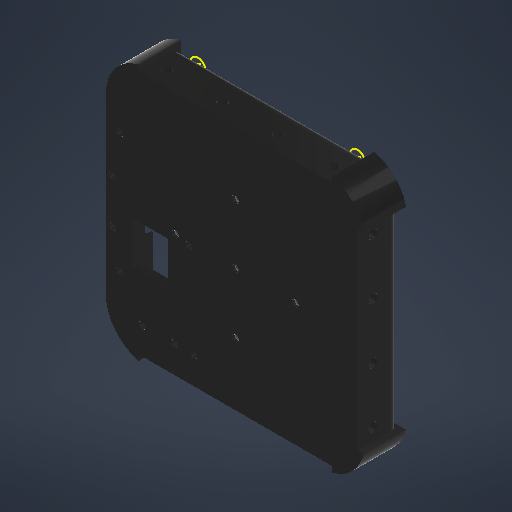
# Autodesk Inventor part: battery_spacer
Saved by Autodesk Inventor 2026.1 (Build 301233000, 233)
## iProperties
Created: 2026-05-19
Part Number: battery_spacer
Material: ABS Plastic
Document SubType Name: Modeling
Designer: aaron
Density: 1.06 g/cm^3
Appearance: Smooth - White
Author: aaron
Autodesk Inventor part; units mm, degrees
ref_plane "YZ Plane" through (0, 0, 0) normal (1, 0, 0) x (0, 1, 0)
ref_plane "XZ Plane" through (0, 0, 0) normal (0, 1, 0) x (-1, 0, 0)
ref_plane "XY Plane" through (0, 0, 0) normal (0, 0, 1) x (1, 0, 0)
sketch "Sketch1" plane through (0, 0, 0) normal (0, 0, 1) x (1, 0, 0)
  circle A0 centre (-25.1008, -25.8499) radius 6
  circle A1 centre (30.8992, 30.1501) radius 6
  circle A2 centre (56.8992, 30.1501) radius 2.15
  circle A3 centre (-51.1008, -25.8499) radius 2.15
  circle A4 centre (-51.1008, 30.1501) radius 2.15
  circle A5 centre (56.8992, -25.8499) radius 2.15
  circle A6 centre (30.8992, 56.1501) radius 2.15
  circle A7 centre (-25.1008, -51.8499) radius 2.15
  circle A8 centre (-25.1008, 56.1501) radius 2.15
  circle A9 centre (30.8992, -51.8499) radius 2.15
  line L0 (48.0316, -57.806) -> (48.0316, -55.1499)
  arc A10 (48.0316, -57.806) -> (62.8553, -42.9824) centre (43.3992, -38.3499) ccw
  line L1 (60.1992, -42.9824) -> (62.8553, -42.9824)
  line L2 (60.1992, -42.9824) -> (60.1992, 47.2825)
  line L3 (62.8553, 47.2825) -> (60.1992, 47.2825)
  arc A11 (62.8553, 47.2825) -> (48.0316, 62.1062) centre (43.3992, 42.6501) ccw
  line L4 (48.0316, 59.4501) -> (48.0316, 62.1062)
  line L5 (48.0316, 59.4501) -> (-42.2333, 59.4501)
  line L6 (-42.2333, 62.1062) -> (-42.2333, 59.4501)
  arc A12 (-42.2333, 62.1062) -> (-57.6008, 42.6501) centre (-37.6008, 42.6501) ccw
  line L7 (-57.6008, -38.3499) -> (-57.6008, 42.6501)
  arc A13 (-57.6008, -38.3499) -> (-42.2333, -57.806) centre (-37.6008, -38.3499) ccw
  line L8 (-42.2333, -55.1499) -> (-42.2333, -57.806)
  line L9 (-42.2333, -55.1499) -> (48.0316, -55.1499)
  circle A14 centre (-25.1008, 2.1501) radius 2.15
  circle A15 centre (2.8992, 30.1501) radius 2.15
  circle A16 centre (30.8992, 2.1501) radius 2.15
  circle A17 centre (2.8992, -25.8499) radius 2.15
  circle A18 centre (2.8992, 2.1501) radius 2.15
  circle A19 centre (-39.1008, -39.8499) radius 13.125
  circle A20 centre (-11.1008, -39.8499) radius 13.125
  circle A21 centre (-11.1008, 16.1501) radius 13.125
  circle A22 centre (44.8992, 16.1501) radius 13.125
  circle A23 centre (44.8992, -11.8499) radius 13.125
  circle A24 centre (44.8992, -39.8499) radius 13.125
  circle A25 centre (16.8992, 44.1501) radius 13.125
  circle A26 centre (16.8992, 16.1501) radius 13.125
  circle A27 centre (16.8992, -11.8499) radius 13.125
  circle A28 centre (16.8992, -39.8499) radius 13.125
  circle A29 centre (-11.1008, 44.1501) radius 13.125
  circle A30 centre (-11.1008, -11.8499) radius 13.125
  circle A31 centre (-39.1008, 44.1501) radius 13.125
  circle A32 centre (-39.1008, -11.8499) radius 13.125
  circle A33 centre (44.8992, 44.1501) radius 13.125
  circle A34 centre (30.8992, -25.8499) radius 6
  circle A35 centre (-25.1008, 30.1501) radius 6
  point P0 (0, 0)
  point P1 (54.9491, 53.8254)
  constraints: 36 centre point, 20 end point, 8 point on circle
extrude "Extrusion1" add sketch "Sketch1" along normal blind 19.82 contours A0 | A1 | A2 | A3 | A4 | A5 | A6 | A7 | A8 | A9 | L0 L9 L8 A13 L7 A12 L6 L5 L4 A11 L3 L2 L1 A10 | A14 | A15 | A16 | A17 | A18 | A19 | A20 | A21 | A22 | A23 | A24 | A25 | A26 | A27 | A28 | A29 | A30 | A31 | A32 | A33 | A34 | A35
fillet "Fillet1" radius 5 3 edges at (2.8992, 59.4501, 0) (2.8992, -55.1499, 0) (60.1992, 2.1501, 0)
sketch "Sketch2" plane through (-42.2333, 59.4501, 19.82) normal (0, 1, 0) x (1, 0, 0)
  circle A0 centre (6.1325, 7) radius 1.65 projected
  circle A1 centre (32.1325, 7) radius 1.65 projected
  circle A2 centre (58.1325, 7) radius 1.65 projected
  circle A3 centre (84.1325, 7) radius 1.65 projected
  circle A4 centre (6.1325, 7) radius 2.15
  circle A5 centre (32.1325, 7) radius 2.15
  circle A6 centre (58.1325, 7) radius 2.15
  circle A7 centre (84.1325, 7) radius 2.15
  point P0 (42.2333, 19.82)
  dimension "d3" = 4.3
  dimension "d4" = 4.3
  dimension "d5" = 4.3
  dimension "d6" = 4.3
  constraints: 4 centre point, 4 coincident
  measures "d3" diameter of A4
  measures "d4" diameter of A5
  measures "d5" diameter of A6
  measures "d6" diameter of A7
sketch "Sketch3" plane through (60.1992, -42.9824, 19.82) normal (1, 0, 0) x (0, 0, -1)
  circle A0 centre (7, 84.1125) radius 1.65 projected
  circle A1 centre (7, 58.1125) radius 1.65 projected
  circle A2 centre (7, 32.1125) radius 1.65 projected
  circle A3 centre (7, 6.1125) radius 1.65 projected
  circle A4 centre (7, 6.1125) radius 2.15
  circle A5 centre (7, 32.1125) radius 2.15
  circle A6 centre (7, 58.1125) radius 2.15
  circle A7 centre (7, 84.1125) radius 2.15
  point P0 (19.82, 42.9824)
  dimension "d11" = 4.3
  dimension "d12" = 4.3
  dimension "d13" = 4.3
  dimension "d14" = 4.3
  constraints: 4 centre point, 4 coincident
  measures "d11" diameter of A4
  measures "d12" diameter of A5
  measures "d13" diameter of A6
  measures "d14" diameter of A7
extrude "Extrusion2" cut sketch "Sketch2" against normal blind 10 contours A0 | A1 | A2 | A3 | A4 | A5 | A6 | A7
sketch "Sketch4" plane through (-42.2333, -55.1499, 19.82) normal (0, -1, 0) x (1, 0, 0)
  circle A0 centre (32.1325, -7) radius 2.15 projected
  circle A1 centre (6.1325, -7) radius 2.15 projected
  circle A2 centre (58.1325, -7) radius 2.15 projected
  circle A3 centre (84.1325, -7) radius 2.15 projected
  point P0 (42.2333, -19.82)
extrude "Extrusion3" cut sketch "Sketch4" against normal blind 10
extrude "Extrusion4" cut sketch "Sketch3" against normal blind 10 contours A0 | A1 | A2 | A3 | A4 | A5 | A6 | A7
sketch "Sketch5" plane through (0, 0, 0) normal (0, 0, -1) x (-1, 0, 0)
  line L0 (39.6008, 53.4501) -> (-48.1992, 53.4501)
  line L1 (-54.1992, 47.4501) -> (-54.1992, -43.1499)
  line L2 (-48.1992, -49.1499) -> (39.6008, -49.1499)
  line L3 (45.6008, -43.1499) -> (45.6008, 47.4501)
  line L4 (57.6008, 42.6501) -> (57.6008, -38.3499) projected
  line L5 (42.2333, 59.4501) -> (-48.0316, 59.4501) projected
  line L6 (-48.0316, -55.1499) -> (42.2333, -55.1499) projected
  line L7 (-60.1992, 47.2825) -> (-60.1992, -42.9824) projected
  arc A0 (45.6008, 47.4501) -> (39.6008, 53.4501) centre (39.6008, 47.4501) ccw
  arc A1 (39.6008, -49.1499) -> (45.6008, -43.1499) centre (39.6008, -43.1499) ccw
  arc A2 (-54.1992, -43.1499) -> (-48.1992, -49.1499) centre (-48.1992, -43.1499) ccw
  arc A3 (-48.1992, 53.4501) -> (-54.1992, 47.4501) centre (-48.1992, 47.4501) ccw
  point P0 (0, 0)
  dimension "d17" = 12
  dimension "d18" = 6
  dimension "d19" = 6
  dimension "d20" = 6
  dimension "d21" = 6
  constraints: 8 end point, 8 point on circle, 8 tangent, 4 centre point, 3 equal radius, 2 parallel, 1 horizontal, 1 perpendicular
  measures "d17" distance between parallel lines of L4 L3
  measures "d18" distance between parallel lines of L5 L0
  measures "d19" distance between parallel lines of L6 L2
  measures "d20" distance between parallel lines of L7 L1
  measures "d21" radius of A0
extrude "Extrusion5" cut sketch "Sketch5" against normal blind 16.82
sketch "Sketch6" plane through (0, 0, 0) normal (0, 0, -1) x (-1, 0, 0)
  circle A0 centre (51.1008, -25.8699) radius 2.15 projected
  circle A1 centre (51.1008, 30.1301) radius 2.15 projected
  circle A2 centre (-2.8992, 2.1301) radius 2.15 projected
  circle A3 centre (25.1008, 2.1301) radius 2.15 projected
  circle A4 centre (-2.8992, -25.8699) radius 2.15 projected
  circle A5 centre (-2.8992, 30.1301) radius 2.15 projected
  circle A6 centre (-30.8992, 2.1301) radius 2.15 construction
  circle A7 centre (-30.8992, 2.1301) radius 2.15 projected
  circle A8 centre (51.1008, 30.1301) radius 1.65
  circle A9 centre (51.1008, -25.8699) radius 1.65
  circle A10 centre (25.1008, 2.1301) radius 1.65
  circle A11 centre (-2.8992, 30.1301) radius 1.65
  circle A12 centre (-2.8992, 2.1301) radius 1.65
  circle A13 centre (-30.8992, 2.1301) radius 1.65
  circle A14 centre (-2.8992, -25.8699) radius 1.65
  point P0 (0, 0)
  dimension "d24" = 3.3
  dimension "d25" = 3.3
  dimension "d26" = 3.3
  dimension "d27" = 3.3
  dimension "d28" = 3.3
  dimension "d29" = 3.3
  dimension "d30" = 3.3
  constraints: 7 centre point, 7 coincident
  measures "d24" diameter of A8
  measures "d25" diameter of A9
  measures "d26" diameter of A10
  measures "d27" diameter of A11
  measures "d28" diameter of A12
  measures "d29" diameter of A13
  measures "d30" diameter of A14
extrude "Extrusion6" cut sketch "Sketch6" against normal through all contours A8 | A9 | A10 | A11 | A12 | A13 | A14
chamfer "Chamfer1" distance 1.8 angle 45 5 edges at (-23.4508, 2.1301, 16.82) (4.5492, 2.1301, 16.82) (4.5492, -25.8699, 16.82) (32.5492, 2.1301, 16.82) (4.5492, 30.1301, 16.82)
sketch "Sketch7" plane through (-57.6008, -38.3499, 0) normal (-1, 0, 0) x (0, 0, 1)
  line L0 (0, 0.9717) -> (-14.73, 0.9717) construction
  line L1 (0, 0.9717) -> (-14.73, 0.9717) construction
  line L2 (-14.73, 55.9717) -> (0, 55.9717) construction
  line L3 (0, 0.9717) -> (12, 0.9717) construction
  line L4 (12, 0.9717) -> (12, 55.9717) construction
  line L5 (12, 55.9717) -> (0, 55.9717) construction
  line L6 (0, 55.9717) -> (0, 0.9717) construction
  line L7 (12, 0.9717) -> (0, 0.9717)
  line L8 (0, 0.9717) -> (0, 55.9717)
  line L9 (0, 55.9717) -> (12, 55.9717)
  line L10 (12, 55.9717) -> (12, 0.9717)
  line L11 (0, 81) -> (0, 0) projected
  point P0 (0, 38.3499)
  dimension "d38" = 12
  constraints: 16 end point, 4 parallel, 2 horizontal, 2 perpendicular
  measures "d38" distance between parallel lines of L4 L11
extrude "Extrusion7" cut sketch "Sketch7" against normal blind 11.35
sketch "Sketch8" plane through (-57.6008, -38.3499, 19.82) normal (-1, 0, 0) x (0, 0, 1)
  circle A0 centre (-11.895, 63.8967) radius 7.925
  line L0 (-19.82, 81) -> (-19.82, 55.9717) projected
  line L1 (-19.82, 55.9717) -> (-7.82, 55.9717) projected
  point P0 (-19.82, 38.3499)
  point P1 (-19.82, 63.8967)
  point P2 (-11.895, 55.9717)
  dimension "d39" = 15.85
  constraints: 2 tangent, 1 centre point
  measures "d39" diameter of A0
extrude "Extrusion8" cut sketch "Sketch8" against normal blind 20
sketch "Sketch9" plane through (-57.6008, -37.3782, 12) normal (0, 0, -1) x (-1, 0, 0)
  line L0 (2.9142, 50.8583) -> (-29.0224, 50.8583)
  line L1 (-29.0224, 50.8583) -> (-29.0224, 25.1583)
  line L2 (-29.0224, 25.1583) -> (2.9142, 25.1583)
  line L3 (2.9142, 25.1583) -> (2.9142, 50.8583)
  circle A0 centre (-6.5, 11.5083) radius 1.65 projected
  point P0 (-57.6008, 37.3782)
  dimension "d42" = 25.7
  dimension "d43" = 12
  constraints: 8 end point, 2 parallel, 1 horizontal, 1 perpendicular
  measures "d42" distance of L2.end L0.start
  measures "d43" distance edge to line of A0 L2
extrude "Extrusion9" cut sketch "Sketch9" along normal mid plane 3.4 contours L3 L2 L1 L0
sketch "Sketch10" plane through (-57.6008, -37.3782, 13.7) normal (0, 0, -1) x (-1, 0, 0)
  line L0 (0, 50.8583) -> (0, 25.1583) projected
  line L1 (-12, 50.8583) -> (0, 50.8583) projected
  line L2 (-12, 25.1583) -> (-12, 50.8583) projected
  line L3 (0, 25.1583) -> (-12, 25.1583) projected
  point P0 (-57.6008, 37.3782)
extrude "Extrusion10" cut sketch "Sketch10" along normal through all
sketch "Sketch11" plane through (-57.6008, -37.3782, 13.7) normal (0, 0, -1) x (-1, 0, 0)
  circle A0 centre (-3, 48.2583) radius 1.65
  line L0 (0, 25.1583) -> (-11.35, 25.1583) projected
  line L1 (-11.35, 50.8583) -> (0, 50.8583) projected
  line L2 (-7.8548, 38.0083) -> (4.7845, 38.0083)
  circle A1 centre (-3, 27.7583) radius 1.65
  line L3 (0, 50.8583) -> (0, 25.1583) projected
  point P0 (-57.6008, 37.3782)
  dimension "d48" = 25.7
  dimension "d49" = 2.6
  dimension "d50" = 12.85
  dimension "d51" = 3
  dimension "d52" = 3.3
  constraints: 2 centre point, 2 end point, 1 horizontal, 1 symmetric about line, 1 other
  measures "d48" distance between parallel lines of L0 L1
  measures "d49" distance from line of L1 A0.centre
  measures "d50" distance between parallel lines of L1 L2
  measures "d51" distance from line of L3 A0.centre
  measures "d52" diameter of A0
extrude "Extrusion11" cut sketch "Sketch11" against normal through all
sketch "Sketch12" plane through (0, 0, 0) normal (0, 0, -1) x (-1, 0, 0)
  line L0 (60.2502, 30.5543) -> (43.0024, 30.5543)
  line L1 (43.0024, 30.5543) -> (43.0024, -35.237)
  line L2 (43.0024, -35.237) -> (60.2502, -35.237)
  line L3 (60.2502, -35.237) -> (60.2502, 30.5543)
  point P0 (0, 0)
  constraints: 8 end point, 2 parallel, 1 horizontal, 1 perpendicular
extrude "Extrusion12" cut sketch "Sketch12" against normal blind 10
sketch "Sketch13" plane through (-57.6008, -37.3782, 13.7) normal (0, 0, -1) x (-1, 0, 0)
  line L0 (0, 50.8583) -> (0, 25.1583) projected
  line L1 (0, 43.0833) -> (-10, 43.0833)
  line L2 (-10, 43.0833) -> (-10, 32.9333)
  line L3 (-10, 32.9333) -> (0, 32.9333)
  line L4 (0, 32.9333) -> (0, 43.0833)
  line L5 (0, 25.1583) -> (-11.35, 25.1583) projected
  line L6 (-11.35, 50.8583) -> (0, 50.8583) projected
  line L7 (-6.1596, 43.0833) -> (-6.1596, 50.8583)
  line L8 (-6.1596, 32.9333) -> (-6.1596, 25.1583)
  point P0 (-57.6008, 37.3782)
  point P1 (0, 32.9333)
  dimension "d57" = 25.7
  dimension "d58" = 10.15
  dimension "d59" = 10
  constraints: 12 end point, 7 point on line, 2 parallel, 2 perpendicular, 1 collinear, 1 horizontal
  measures "d57" distance between parallel lines of L5 L6
  measures "d58" distance of L1.end L2.end
  measures "d59" distance of L2.end L3.end
extrude "Extrusion13" cut sketch "Sketch13" against normal blind 4 contours L0 L3 L2 L1
chamfer "Chamfer2" distance 1.8 angle 45 1 edges at (-49.4508, -25.8699, 12)
sketch "Sketch14" plane through (0, 0, 16.82) normal (0, 0, -1) x (-1, 0, 0)
  line L0 (45.6008, -12.2199) -> (45.6008, 13.4801) projected
  line L1 (45.6008, -1.5499) -> (28.6008, -1.5499)
  line L2 (28.6008, -1.5499) -> (28.6008, -21.5499)
  line L3 (28.6008, -21.5499) -> (45.6008, -21.5499)
  line L4 (45.6008, -21.5499) -> (45.6008, -1.5499)
  line L5 (-48.0316, 54.4501) -> (42.2333, 54.4501) projected
  line L6 (42.2333, 59.4501) -> (-48.0316, 59.4501) projected
  point P0 (0, 0)
  dimension "d65" = 20
  dimension "d66" = 17
  dimension "d70" = 61
  constraints: 8 end point, 2 parallel, 1 horizontal, 1 perpendicular, 1 point on line
  measures "d65" distance of L1.end L2.end
  measures "d66" distance of L1.start L1.end
  measures "d70" distance between parallel lines of L6 L1
extrude "Extrusion14" cut sketch "Sketch14" against normal through all
sketch "Sketch15" plane through (0, 0, 16.82) normal (0, 0, -1) x (-1, 0, 0)
  circle A0 centre (40.6008, -42.5499) radius 3.5
  circle A1 centre (25.6008, -42.5499) radius 3.5
  line L0 (38.6008, -30.5499) -> (13.6008, -30.5499)
  line L1 (13.6008, -30.5499) -> (13.6008, -32.5499)
  line L2 (13.6008, -32.5499) -> (38.6008, -32.5499)
  line L3 (38.6008, -32.5499) -> (38.6008, -30.5499)
  circle A2 centre (18.8508, 0.6301) radius 3.5
  circle A3 centre (16.6008, -42.5499) radius 3.5
  line L4 (16.0008, 13.4801) -> (13.0008, 13.4801)
  line L5 (13.0008, 13.4801) -> (13.0008, 7.4801)
  line L6 (13.0008, 7.4801) -> (16.0008, 7.4801)
  line L7 (16.0008, 7.4801) -> (16.0008, 13.4801)
  line L8 (16.0008, -6.2199) -> (13.0008, -6.2199)
  line L9 (13.0008, -6.2199) -> (13.0008, -12.2199)
  line L10 (13.0008, -12.2199) -> (16.0008, -12.2199)
  line L11 (16.0008, -12.2199) -> (16.0008, -6.2199)
  line L12 (40.6008, -42.5499) -> (25.6008, -42.5499)
  line L13 (45.6008, -21.5499) -> (28.6008, -21.5499) projected
  line L14 (28.6008, -21.5499) -> (28.6008, -1.5499) projected
  line L15 (57.6008, -12.2199) -> (46.2508, -12.2199) projected
  line L16 (46.2508, 13.4801) -> (57.6008, 13.4801) projected
  line L17 (57.6008, 13.4801) -> (57.6008, 5.7051) projected
  line L18 (57.6008, -4.4449) -> (57.6008, -12.2199) projected
  circle A4 centre (25.1008, 2.1301) radius 3.45 projected
  point P0 (0, 0)
  point P1 (22.3106, 0.101)
  point P2 (21.6936, 2.6718)
  dimension "d71" = 15
  dimension "d72" = 7
  dimension "d73" = 7
  dimension "d74" = 7
  dimension "d75" = 12
  dimension "d76" = 21
  dimension "d77" = 25
  dimension "d78" = 2
  dimension "d80" = 9
  dimension "d81" = 0
  dimension "d82" = 9
  dimension "d83" = 25.7
  dimension "d84" = 12.85
  dimension "d85" = 7
  dimension "d86" = 41.6
  dimension "d87" = 3
  dimension "d88" = 0
  dimension "d89" = 0
  dimension "d90" = 6
  dimension "d91" = 6
  dimension "d92" = 38.75
  dimension "d103" = 10
  constraints: 26 end point, 7 parallel, 4 centre point, 4 horizontal, 3 perpendicular, 2 point on line
  measures "d71" distance of L12.start L12.end
  measures "d72" diameter of A0
  measures "d73" diameter of A1
  measures "d74" diameter of A3
  measures "d75" distance from line of L14 L12.start
  measures "d76" distance between parallel lines of L13 L12
  measures "d77" distance of L0.start L0.end
  measures "d78" distance between parallel lines of L2 L0
  measures "d80" distance between parallel lines of L13 L0
  measures "d81" distance from line of L12 A3.centre
  measures "d82" distance of L12.end A3.centre
  measures "d83" distance between parallel lines of L15 L16
  measures "d84" distance from line of L16 A2.centre
  measures "d85" diameter of A2
  measures "d86" distance between parallel lines of L7 L17
  measures "d87" distance between parallel lines of L7 L5
  measures "d88" distance between parallel lines of L16 L4
  measures "d89" distance between parallel lines of L10 L15
  measures "d90" distance of L4.end L5.end
  measures "d91" distance of L8.end L9.end
  measures "d92" distance from line of L18 A2.centre
  measures "d103" distance between parallel lines of L3 L14
extrude "Extrusion15" add sketch "Sketch15" along normal up to surface (3.12 mm away) contours A0 | A1 | L3 L2 L1 L0 | A4 A2 | A3 | L7 L6 L5 L4 | L11 L10 L9 L8 picked at (17.5632, 0.3211)
sketch "Sketch16" plane through (-18.8508, 0.6301, 13.7) normal (0, 0, -1) x (-0.9723873, 0.233373, 0)
  arc A0 (3.2408, 1.3219) -> (3.2408, -1.3219) centre (0, 0) ccw projected
  circle A1 centre (-12.2649, -41.4626) radius 3.5 projected
  circle A2 centre (-3.5134, -43.563) radius 3.5 projected
  circle A3 centre (11.0724, -47.0635) radius 3.5 projected
  circle A4 centre (11.0724, -47.0635) radius 1.65
  circle A5 centre (-3.5134, -43.563) radius 1.65
  circle A6 centre (-12.2649, -41.4626) radius 1.65
  circle A7 centre (0, 0) radius 1.65
  point P0 (-18.4774, 3.7866)
  dimension "d95" = 3.3
  dimension "d96" = 3.3
  dimension "d97" = 3.3
  dimension "d98" = 3.3
  constraints: 4 centre point, 4 coincident
  measures "d95" diameter of A7
  measures "d96" diameter of A4
  measures "d97" diameter of A5
  measures "d98" diameter of A6
extrude "Extrusion16" cut sketch "Sketch16" against normal through all contours A4 | A5 | A6 | A7
sketch "Sketch17" plane through (-13.0008, 13.4801, 13.7) normal (0, 0, -1) x (-1, 0, 0)
  line L0 (3, 0) -> (0, 0) projected
  line L1 (0, 0) -> (0, -6) projected
  line L2 (0, -6) -> (3, -6) projected
  line L3 (3, -6) -> (3, 0) projected
  line L4 (3, -19.7) -> (0, -19.7) projected
  line L5 (0, -19.7) -> (0, -25.7) projected
  line L6 (0, -25.7) -> (3, -25.7) projected
  line L7 (3, -25.7) -> (3, -19.7) projected
  point P0 (-13.0008, -13.4801)
extrude "Extrusion17" add sketch "Sketch17" along normal blind 1.6
chamfer "Chamfer3" distance 1 angle 45 10 edges at (-13.0008, 10.4801, 16.82) (-13.0008, -9.2199, 16.82) (-16.0008, -9.2199, 16.82) (-16.0008, 10.4801, 16.82) (-15.4475, -0.1867, 16.82) (-13.1008, -42.5499, 16.82) (-22.1008, -42.5499, 16.82) (-37.1008, -42.5499, 16.82) (-26.1008, -30.5499, 16.82) (-26.1008, -32.5499, 16.82)
sketch "Sketch18" plane through (-57.6008, -38.3499, 19.82) normal (-1, 0, 0) x (0, 0, 1)
  circle A0 centre (-3.5, 3) radius 1.65
  circle A1 centre (-3.5, 55) radius 1.65
  line L0 (0, 81) -> (0, 0) projected
  line L1 (-19.82, 0) -> (0, 0) projected
  point P0 (-19.82, 38.3499)
  dimension "d107" = 3.3
  dimension "d108" = 3.3
  dimension "d109" = 3.5
  dimension "d110" = 3.5
  dimension "d111" = 3
  dimension "d112" = 52
  constraints: 2 centre point
  measures "d107" diameter of A0
  measures "d108" diameter of A1
  measures "d109" distance from line of L0 A1.centre
  measures "d110" distance from line of L0 A0.centre
  measures "d111" distance from line of L1 A0.centre
  measures "d112" distance of A0.centre A1.centre
extrude "Extrusion18" cut sketch "Sketch18" against normal blind 8
sketch "Sketch19" plane through (0, 0, 0) normal (0, 0, -1) x (-1, 0, 0)
  circle A0 centre (34.3906, 55.3699) radius 3.6 projected
  circle A1 centre (-40.1744, 55.38) radius 3.6 projected
  circle A2 centre (34.376, -51.1199) radius 3.6 projected
  circle A3 centre (-40.1889, -51.1097) radius 3.6 projected
  point P0 (0, 0)
equation "\"d50\" = 0.5 * d48"
equation "\"d73\" = d72"
equation "\"d74\" = d72"
equation "\"d84\" = 0.5 * d83"
equation "\"d96\" = d95"
equation "\"d97\" = d95"
equation "\"d98\" = d95"
equation "\"d109\" = d110"
body "Solid1"
